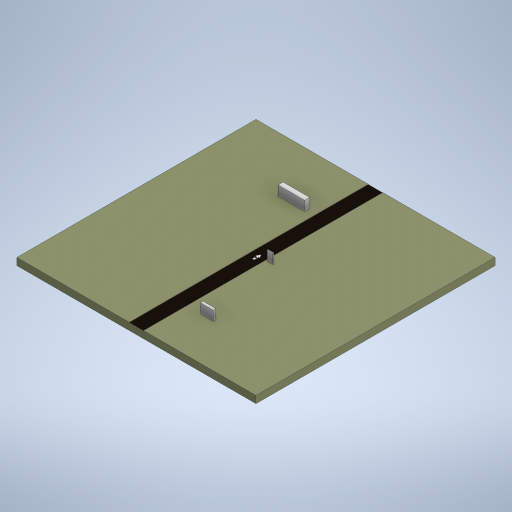
# Autodesk Inventor part: forest1
Saved by Autodesk Inventor 2023 (Build 270158000, 158)
## iProperties
Created: 2022-11-04
Part Number: forest1
Material: Generic
Document SubType Name: Modeling
Designer: derm
Density: 1 g/cm^3
Appearance: Default
Author: derm
Autodesk Inventor part; units mm, degrees
ref_plane "YZ Plane" through (0, 0, 0) normal (1, 0, 0) x (0, 1, 0)
ref_plane "XZ Plane" through (0, 0, 0) normal (0, 1, 0) x (-1, 0, 0)
ref_plane "XY Plane" through (0, 0, 0) normal (0, 0, 1) x (1, 0, 0)
sketch "Sketch1" plane through (0, 0, 0) normal (0, 1, 0) x (-1, 0, 0)
  line L0 (-50000, 50000) -> (50000, 50000)
  line L1 (50000, 50000) -> (50000, -50000)
  line L2 (50000, -50000) -> (-50000, -50000)
  line L3 (-50000, -50000) -> (-50000, 50000)
  line L4 (-50000, 50000) -> (50000, -50000) construction
  line L5 (50000, 50000) -> (-50000, -50000) construction
  point P0 (0, 0)
  dimension "d0" = 100000
  dimension "d1" = 100000
  constraints: 12 end point, 2 midpoint, 2 parallel, 1 horizontal, 1 perpendicular
  measures "d0" distance of L0.end L1.end
  measures "d1" distance of L1.end L2.end
extrude "Extrusion1" add sketch "Sketch1" against normal blind 3000
sketch "Sketch2" plane through (0, 0, 0) normal (0, 1, 0) x (1, 0, 0)
  line L0 (-50000, 50000) -> (50000, 50000) projected
  line L1 (3000, -50000) -> (-3000, -50000)
  line L2 (-3000, -50000) -> (-3000, 50000)
  line L3 (-3000, 50000) -> (3000, 50000)
  line L4 (3000, 50000) -> (3000, -50000)
  line L5 (3000, -50000) -> (-3000, 50000) construction
  line L6 (-3000, -50000) -> (3000, 50000) construction
  point P0 (0, 0)
  dimension "d4" = 6000
  constraints: 12 end point, 2 midpoint, 2 parallel, 1 horizontal, 1 perpendicular, 1 point on line
  measures "d4" distance between parallel lines of L4 L2
extrude "Extrusion2" cut sketch "Sketch2" against normal blind 100
sketch "Sketch3" plane through (0, 0, 0) normal (0, 1, 0) x (1, 0, 0)
  line L0 (3000, 50000) -> (3000, -50000) projected
  line L1 (3000, -50000) -> (50000, -50000) projected
  line L2 (50000, -50000) -> (50000, 50000) projected
  line L3 (50000, 50000) -> (3000, 50000) projected
  circle A0 centre (-5162.0769, 2791.8732) radius 250
  circle A1 centre (3448.1949, 3556.0433) radius 250
  point P0 (0, 0)
  dimension "d7" = 500
  dimension "d8" = 500
  constraints: 2 centre point
  measures "d7" diameter of A0
  measures "d8" diameter of A1
extrude "Extrusion3" [suppressed]
pattern_linear "Rectangular Pattern1" [suppressed]
pattern_linear "Rectangular Pattern2" [suppressed]
sketch "Sketch4" plane through (0, 0, 0) normal (0, 1, 0) x (1, 0, 0)
  line L0 (3656.3304, 1373.5123) -> (6095.1457, 1373.5123)
  line L1 (6095.1457, 1373.5123) -> (6095.1457, 1000)
  line L2 (6095.1457, 1000) -> (3656.3304, 1000)
  line L3 (3656.3304, 1000) -> (3656.3304, 1373.5123)
  line L4 (-17614.0817, 28959.908) -> (-6502.6944, 28959.908)
  line L5 (-6502.6944, 28959.908) -> (-6502.6944, 26841.9015)
  line L6 (-6502.6944, 26841.9015) -> (-17614.0817, 26841.9015)
  line L7 (-17614.0817, 26841.9015) -> (-17614.0817, 28959.908)
  line L8 (8740.9777, -30936.9942) -> (14162.228, -30936.9942)
  line L9 (14162.228, -30936.9942) -> (14162.228, -32058.6321)
  line L10 (14162.228, -32058.6321) -> (8740.9777, -32058.6321)
  line L11 (8740.9777, -32058.6321) -> (8740.9777, -30936.9942)
  point P0 (0, 0)
  dimension "d17" = 1000
  constraints: 24 end point, 6 parallel, 3 horizontal, 3 perpendicular
  measures "d17" distance from line of point (0, 0) L2
extrude "Extrusion4" add sketch "Sketch4" along normal blind 4000
sketch "Sketch5" plane through (0, -100, 0) normal (0, 1, 0) x (1, 0, 0)
  line L0 (-437.7268, -1196.5922) -> (437.7268, -1196.5922)
  line L1 (437.7268, -1196.5922) -> (437.7268, 1196.5922)
  line L2 (437.7268, 1196.5922) -> (-437.7268, 1196.5922)
  line L3 (-437.7268, 1196.5922) -> (-437.7268, -1196.5922)
  line L4 (-437.7268, -1196.5922) -> (437.7268, 1196.5922) construction
  line L5 (437.7268, -1196.5922) -> (-437.7268, 1196.5922) construction
  line L6 (0, 2199.5256) -> (868.5658, 695.1255)
  line L7 (868.5658, 695.1255) -> (-868.5658, 695.1255)
  line L8 (-868.5658, 695.1255) -> (0, 2199.5256)
  circle A0 centre (0, 0) radius 250
  point P0 (0, 1196.5922)
  point P1 (437.7268, 695.1255)
  point P2 (-437.7268, 695.1255)
  dimension "d23" = 500
  constraints: 18 end point, 3 midpoint, 2 parallel, 1 centre point, 1 coincident, 1 horizontal, 1 perpendicular, 9 other
  measures "d23" diameter of A0
extrude "Extrusion5" cut sketch "Sketch5" against normal blind 1
body "Solid1"
